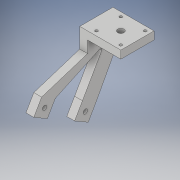
# Autodesk Inventor part: Stepper_Face
Saved by Autodesk Inventor 2019 (Build 230136000, 136)
## iProperties
Created: 2019-07-06
Part Number: Stepper_Face
Material: Generic
Document SubType Name: Modeling
Designer: Jorian Brusind
Density: 1 g/cm^3
Appearance: Default
Author: Jorian Brusind
Autodesk Inventor part; units mm, degrees
ref_plane "YZ Plane" through (0, 0, 0) normal (1, 0, 0) x (0, 1, 0)
ref_plane "XZ Plane" through (0, 0, 0) normal (0, 1, 0) x (-1, 0, 0)
ref_plane "XY Plane" through (0, 0, 0) normal (0, 0, 1) x (1, 0, 0)
sketch "Sketch1" plane through (0, 0, 0) normal (0, 1, 0) x (-1, 0, 0)
  line L0 (0, 0) -> (52.3, 0)
  line L1 (52.3, 0) -> (52.3, -42.3)
  line L2 (52.3, -42.3) -> (0, -42.3)
  line L3 (0, -42.3) -> (0, 0)
  dimension "d0" = 52.3
  dimension "d1" = 42.3
  constraints: 8 end point, 2 parallel, 1 horizontal, 1 perpendicular
  measures "d0" distance of L1.end L2.end
  measures "d1" distance of L0.end L1.end
extrude "Extrusion1" add sketch "Sketch1" along normal blind 10
sketch "Sketch2" plane through (0, 0, 0) normal (0, -1, 0) x (1, 0, 0)
  line L0 (-52.3, 0) -> (0, 0) projected
  line L1 (-52.3, 0) -> (-42.3, 0)
  line L2 (-42.3, 0) -> (-42.3, -42.3)
  line L3 (-42.3, -42.3) -> (-52.3, -42.3)
  line L4 (-52.3, -42.3) -> (-52.3, 0)
  dimension "d4" = 10
  dimension "d5" = 42.3
  constraints: 8 end point, 2 parallel, 1 horizontal, 1 perpendicular
  measures "d4" distance of L2.end L3.end
  measures "d5" distance of L1.end L2.end
extrude "Extrusion2" add sketch "Sketch2" along normal blind 15
sketch "Sketch3" plane through (0, 10, 0) normal (0, 1, 0) x (1, 0, 0)
  line L0 (0, 0) -> (0, 5.65)
  line L1 (0, 0) -> (0, 42.3) projected
  line L2 (0, 5.65) -> (-5.65, 5.65)
  circle A0 centre (-5.65, 5.65) radius 1.75
  circle A1 centre (-5.65, 36.65) radius 1.75
  circle A2 centre (-36.65, 5.65) radius 1.75
  circle A3 centre (-36.65, 36.65) radius 1.75
  dimension "d8" = 5.65
  dimension "d9" = 5.65
  dimension "d10" = 3.5
  dimension "d13" = 31
  dimension "d16" = 31
  constraints: 4 centre point, 4 end point, 1 coincident, 1 horizontal, 1 perpendicular, 1 point on line, 1 vertical, 6 other
  measures "d8" distance of L0.start L0.end
  measures "d9" distance of L0.end L2.end
  measures "d10" diameter of A0
  measures "d13" distance of A0.centre A1.centre
  measures "d16" distance of A0.centre A2.centre
extrude "Extrusion3" cut sketch "Sketch3" against normal blind 10
sketch "Sketch4" plane through (0, 10, 0) normal (0, 1, 0) x (1, 0, 0)
  line L0 (0, 42.3) -> (0, 0) projected
  line L1 (0, 21.15) -> (-21.15, 21.15)
  circle A0 centre (-21.15, 21.15) radius 4
  dimension "d21" = 21.15
  dimension "d22" = 8
  constraints: 2 end point, 1 centre point, 1 coincident, 1 horizontal, 1 midpoint
  measures "d21" distance of L1.start L1.end
  measures "d22" diameter of A0
extrude "Extrusion4" cut sketch "Sketch4" against normal blind 10
sketch "Sketch9" plane through (-52.3, 10, -42.3) normal (-1, 0, 0) x (0, 0, 1)
  line L0 (42.3, 0) -> (0, 0) projected
  line L1 (21.15, 0) -> (121.15, 0) construction
  line L2 (42.3, 0) -> (42.3, -25) projected
  line L3 (0, -25) -> (42.3, -25) projected
  line L4 (21.15, 0) -> (21.15, 14.2)
  line L5 (21.15, 14.2) -> (71.15, -72.4025)
  line L6 (21.15, 14.2) -> (121.15, 14.2) construction
  line L7 (71.15, -72.4025) -> (62.4897, -77.4025)
  line L8 (57.4897, -68.7423) -> (74.8103, -58.7423)
  line L9 (74.8103, -58.7423) -> (84.8103, -76.0628)
  line L10 (84.8103, -76.0628) -> (67.4897, -86.0628)
  line L11 (67.4897, -86.0628) -> (57.4897, -68.7423)
  line L12 (57.4897, -68.7423) -> (84.8103, -76.0628) construction
  line L13 (74.8103, -58.7423) -> (67.4897, -86.0628) construction
  line L14 (57.4897, -68.7423) -> (77.4897, -68.7423) construction
  line L15 (71.15, -72.4025) -> (97.1308, -57.4025)
  line L16 (71.15, -72.4025) -> (45.1692, -87.4025)
  line L17 (71.15, -72.4025) -> (101.15, -72.4025) construction
  circle A0 centre (97.1308, -57.4025) radius 2.75
  circle A1 centre (45.1692, -87.4025) radius 2.75
  line L18 (83.4705, -53.7423) -> (100.791, -43.7423)
  line L19 (100.791, -43.7423) -> (110.791, -61.0628)
  line L20 (110.791, -61.0628) -> (93.4705, -71.0628)
  line L21 (93.4705, -71.0628) -> (83.4705, -53.7423)
  line L22 (83.4705, -53.7423) -> (110.791, -61.0628) construction
  line L23 (100.791, -43.7423) -> (93.4705, -71.0628) construction
  line L24 (83.4705, -53.7423) -> (103.4705, -53.7423) construction
  line L25 (0, -10) -> (0, 0) projected
  line L26 (42.3, -25) -> (0, -25) projected
  line L27 (31.509, -83.7423) -> (48.8295, -73.7423)
  line L28 (48.8295, -73.7423) -> (58.8295, -91.0628)
  line L29 (58.8295, -91.0628) -> (41.509, -101.0628)
  line L30 (41.509, -101.0628) -> (31.509, -83.7423)
  line L31 (42.3, -10) -> (42.3, 0) projected
  line L32 (83.4705, -53.7423) -> (21.15, -25)
  line L33 (42.3, -10) -> (42.3, -25) projected
  line L34 (100.791, -43.7423) -> (42.3, -25)
  line L35 (0, -10) -> (0, -25) projected
  line L36 (31.509, -83.7423) -> (0, -25)
  line L37 (48.8295, -73.7423) -> (21.15, -25)
  dimension "d77" = 14.2
  dimension "d78" = 100
  dimension "d79" = 60
  dimension "d80" = 10
  dimension "d81" = 90
  dimension "d82" = 20
  dimension "d83" = 30
  dimension "d84" = 20
  dimension "d85" = 30
  dimension "d86" = 30
  dimension "d87" = 150
  dimension "d88" = 5.5
  dimension "d89" = 5.5
  dimension "d90" = 20
  dimension "d91" = 30
  dimension "d92" = 20
  dimension "d95" = 60
  constraints: 60 end point, 6 midpoint, 5 horizontal, 5 parallel, 4 equal length, 3 perpendicular, 2 centre point, 2 coincident, 1 vertical, 9 other
  measures "d77" distance of L1.start L4.end
  measures "d78" distance of L4.end L5.end
  measures "d79" angle of L5 L6
  measures "d80" distance of L5.end L7.end
  measures "d81" angle of L5 L7
  measures "d82" distance of L8.start L8.end
  measures "d83" angle of L14 L8
  measures "d84" distance of L8.end L9.end
  measures "d85" distance of L5.end L15.end
  measures "d86" distance of L5.end L16.end
  measures "d87" angle of L16 L17
  measures "d88" diameter of A0
  measures "d89" diameter of A1
  measures "d90" distance of L18.start L18.end
  measures "d91" angle of L24 L18
  measures "d92" distance of L18.end L19.end
  measures "d95" distance of L18.start L27.start
extrude "Extrusion9" add sketch "Sketch9" against normal blind 10 contours L3 L37 L27 L36 | L34 L5 L32 L3 | L34 L18 L32 L5 | L27 L28 L29 L30 | L19 L20 L21 L18
fillet "Fillet1" radius 2 1 edges at (-47.3, -15, -21.15)
body "Solid1"
